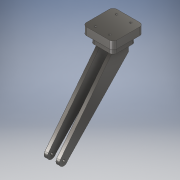
# Autodesk Inventor part: Plate2
Saved by Autodesk Inventor 2018 (Build 220112000, 112)
## iProperties
Created: 2016-06-15
Part Number: Plate2
Material: Polyethylene, High Density
Document SubType Name: Modeling
Designer: Dakota Marin
Density: 0.952 g/cm^3
Appearance: Steel - Polished
Author: Dakota Marin
Autodesk Inventor part; units mm, degrees
ref_plane "XZ Plane" through (0, 0, 0) normal (0, 1, 0) x (-1, 0, 0)
ref_plane "XY Plane" through (0, 0, 0) normal (0, 0, 1) x (1, 0, 0)
sketch "Sketch1" plane through (0, 0, 0) normal (0, 1, 0) x (-1, 0, 0)
  line L0 (-60, -80) -> (60, -80)
  line L1 (80, -60) -> (80, 60)
  line L2 (60, 80) -> (-60, 80)
  line L3 (-80, 60) -> (-80, -60)
  line L4 (-80, -80) -> (80, 80) construction
  line L5 (80, -80) -> (-80, 80) construction
  arc A0 (80, 60) -> (60, 80) centre (60, 60) ccw
  arc A1 (-60, 80) -> (-80, 60) centre (-60, 60) ccw
  arc A2 (-80, -60) -> (-60, -80) centre (-60, -60) ccw
  arc A3 (60, -80) -> (80, -60) centre (60, -60) ccw
  point P0 (0, 0)
  dimension "d0" = 160
  dimension "d1" = 160
  dimension "d2" = 20
  constraints: 12 end point, 8 point on circle, 8 point on line, 8 tangent, 4 centre point, 3 equal radius, 2 midpoint, 2 parallel, 1 horizontal, 1 perpendicular
  measures "d0" distance of L5.start L4.end
  measures "d1" distance of L4.end L5.end
  measures "d2" radius of A0
extrude "Extrusion1" add sketch "Sketch1" along normal blind 40
sketch "Sketch2" plane through (0, 0, 0) normal (0, -1, 0) x (1, 0, 0)
  line L0 (-55, -52.5) -> (55, 52.5) construction
  line L1 (55, -52.5) -> (-55, 52.5) construction
  line L2 (90.8825, 0) -> (-87.3629, 0)
  line L3 (0, 94.4084) -> (0, -106.3516)
  line L4 (-40, -60) -> (40, -60)
  line L5 (60, -40) -> (60, 40)
  line L6 (40, 60) -> (-40, 60)
  line L7 (-60, 40) -> (-60, -40)
  line L8 (-60, -60) -> (60, 60) construction
  line L9 (60, -60) -> (-60, 60) construction
  line L10 (60, 60) -> (41.9971, 60)
  line L11 (60, -60) -> (41.9971, -60)
  line L12 (60, 60) -> (60, 71.6594)
  line L13 (60, -60) -> (60, -69.6689)
  arc A0 (60, 40) -> (40, 60) centre (40, 40) ccw
  arc A1 (-40, 60) -> (-60, 40) centre (-40, 40) ccw
  arc A2 (-60, -40) -> (-40, -60) centre (-40, -40) ccw
  arc A3 (40, -60) -> (60, -40) centre (40, -40) ccw
  point P0 (0, 0)
  dimension "d23" = 60
  dimension "d25" = 60
  dimension "d26" = 20
  constraints: 28 end point, 8 point on circle, 8 point on line, 8 tangent, 5 horizontal, 4 centre point, 4 midpoint, 4 vertical, 3 equal radius, 2 parallel, 1 perpendicular, 1 other
  measures "d23" distance between parallel lines of L2 L10
  measures "d25" distance between parallel lines of L3 L12
  measures "d26" radius of A0
extrude "Extrusion2" add sketch "Sketch2" along normal blind 40
sketch "Sketch3" plane through (0, 40, 0) normal (0, 1, 0) x (1, 0, 0)
  circle A0 centre (-37.5, -55) radius 5
  circle A1 centre (37.5, -55) radius 5
  line L0 (-35.6722, 52.5) -> (-19.5402, 52.5)
  line L1 (0, 83.5001) -> (0, -85.7722)
  line L2 (-75.2069, 0) -> (80.66, 0)
  line L3 (-37.5, -55) -> (37.5, -55)
  line L4 (-37.5, -55) -> (-37.5, -56.2391)
  line L5 (37.5, -55) -> (37.5, -56.2391)
  circle A2 centre (-37.5, 55) radius 5
  circle A3 centre (37.5, 55) radius 5
  point P0 (0, 0)
  dimension "d15" = 37.5
  dimension "d16" = 37.5
  dimension "d17" = 55
  dimension "d20" = 10
  dimension "d21" = 10
  constraints: 12 end point, 4 centre point, 4 vertical, 3 horizontal, 2 symmetric about line, 2 other
  measures "d15" distance between parallel lines of L1 L4
  measures "d16" distance between parallel lines of L1 L5
  measures "d17" distance between parallel lines of L3 L2
  measures "d20" diameter of A2
  measures "d21" diameter of A3
extrude "Extrusion3" cut sketch "Sketch3" against normal blind 6
ref_plane "Work Plane1" through (40, 0, 0) normal (1, 0, 0) x (0, 1, 0)
sketch "Sketch4" plane through (40, 0, 0) normal (1, 0, 0) x (0, 1, 0)
  arc A0 (-396.1638, 317.7429) -> (-418.612, 279.2134) centre (-410, 300) ccw
  circle A1 centre (-410, 300) radius 300
  line L0 (-40, -40) -> (-40, 40) projected
  line L1 (40, 60) -> (40, -60) projected
  line L2 (63.9503, 0) -> (-247.3631, 0)
  line L3 (-410, 300) -> (-214.4005, 300)
  line L4 (-40, -40) -> (-84.0453, -40)
  line L5 (-40, 40) -> (-40, -40)
  line L6 (-40, 40) -> (-396.1638, 317.7429)
  line L7 (-84.0453, -40) -> (-418.612, 279.2134)
  point P0 (0, 0)
  point P1 (-131.6551, 40.5657)
  dimension "d28" = 45
  dimension "d29" = 600
  dimension "d30" = 450
  dimension "d31" = 300
  constraints: 12 end point, 4 horizontal, 2 centre point, 2 point on circle, 1 concentric, 1 tangent, 1 vertical
  measures "d28" diameter of A0
  measures "d29" diameter of A1
  measures "d30" distance from line of A0.centre L1
  measures "d31" distance between parallel lines of L2 L3
extrude "Extrusion4" add sketch "Sketch4" against normal blind 17.5 contours L6 A1 L7 A0 | A1 L6 L0 L2 L7 | L2 L0 L4 L7 picked at (-333.3289, 219.1483)
mirror "Mirror1" about plane through (0, 0, 0) normal (1, 0, 0) of "Extrusion4"
sketch "Sketch5" plane through (60, 0, 40) normal (1, 0, 0) x (0, 0, -1)
  arc A0 (-277.7429, -396.1638) -> (-239.2134, -418.612) centre (-260, -410) ccw projected
  circle A1 centre (-260, -410) radius 7.5
  point P0 (40, 0)
  dimension "d35" = 15
  constraints: 1 centre point, 1 coincident
  measures "d35" diameter of A1
extrude "Extrusion5" cut sketch "Sketch5" against normal through all
body "Solid1"
